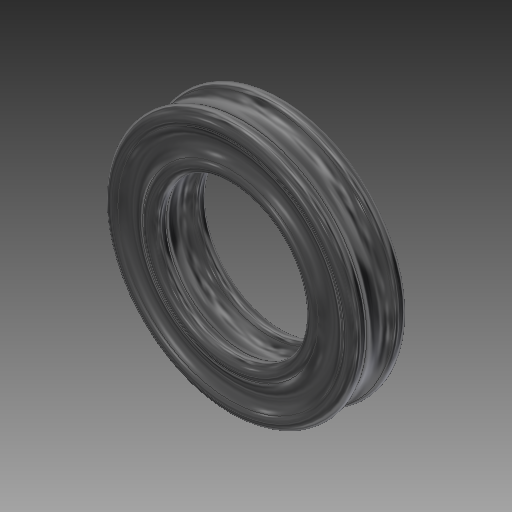
# Autodesk Inventor part: X-Ring 6x2.6
Saved by Autodesk Inventor 2017.3 (Build 213256000, 256)
## iProperties
Created: 2015-08-15
Part Number: X-Ring 6x2.6
Material: Gummi, Silikon
Document SubType Name: Modeling
Designer: rYan
Mass: 0.187427 g
Surface Area: 3.05947 cm^2
Volume: 0.149942 cm^3
Density: 1.25 g/cm^3
Appearance: Gummi - schwarz - Version 1.1
Author: rYan
Autodesk Inventor part; units mm, degrees
ref_plane "YZ Plane" through (0, 0, 0) normal (1, 0, 0) x (0, 1, 0)
ref_plane "XZ Plane" through (0, 0, 0) normal (0, 1, 0) x (-1, 0, 0)
ref_plane "XY Plane" through (0, 0, 0) normal (0, 0, 1) x (1, 0, 0)
sketch "Skizze1" plane through (0, 0, 0) normal (1, 0, 0) x (0, 1, 0)
  arc A0 (-0.63, 5.8857) -> (-1.2127, 5.3385) centre (-0.91, 5.6) ccw
  arc A1 (-0.63, 5.8857) -> (0.63, 5.8857) centre (0, 6.5284) ccw
  arc A2 (1.2127, 5.3385) -> (0.63, 5.8857) centre (0.91, 5.6) ccw
  arc A3 (1.2127, 5.3385) -> (1.2127, 4.1615) centre (1.8936, 4.75) ccw
  arc A4 (0.63, 3.6143) -> (1.2127, 4.1615) centre (0.91, 3.9) ccw
  arc A5 (0.63, 3.6143) -> (-0.63, 3.6143) centre (0, 2.9716) ccw
  arc A6 (-1.2127, 4.1615) -> (-0.63, 3.6143) centre (-0.91, 3.9) ccw
  arc A7 (-1.2127, 4.1615) -> (-1.2127, 5.3385) centre (-1.8936, 4.75) ccw
  line L0 (-0.91, 5.6) -> (0.91, 5.6) construction
  line L1 (0.91, 5.6) -> (0.91, 3.9) construction
  line L2 (0.91, 3.9) -> (-0.91, 3.9) construction
  line L3 (-0.91, 3.9) -> (-0.91, 5.6) construction
  line L4 (0, 7.8341) -> (0, -1.3057) projected
  line L5 (-2.6511, 0) -> (2.6511, 0) construction
  line L6 (0, 5.6) -> (0, 3.9) construction
  line L7 (-0.91, 4.75) -> (0.91, 4.75) construction
  line L8 (-0.91, 5.6) -> (-1.31, 5.6) construction
  line L9 (-0.91, 3.9) -> (-1.31, 3.9) construction
  line L10 (-1.31, 3.9) -> (-1.31, 5.6) construction
  line L11 (-0.91, 5.6) -> (-0.91, 6) construction
  line L12 (-0.91, 3.9) -> (-0.91, 3.5) construction
  line L13 (0.91, 3.9) -> (0.91, 3.5) construction
  line L14 (-0.91, 3.5) -> (0.91, 3.5) construction
  line L15 (0.91, 5.6) -> (1.31, 5.6) construction
  line L16 (0.91, 3.9) -> (1.31, 3.9) construction
  line L17 (-0.91, 6) -> (0.91, 6) construction
  point P0 (0, 0)
  dimension "d0" = 2.5
  dimension "d1" = 7
  dimension "d2" = 2.62
  dimension "d3" = 0.9
  dimension "d4" = 0.4
  constraints: 32 end point, 25 point on circle, 10 tangent, 8 centre point, 7 parallel, 4 horizontal, 4 midpoint, 2 equal radius, 2 vertical, 1 point on line, 3 other
  measures "d0" distance of L12.end L11.end
  measures "d1" diameter of L14 L5
  measures "d2" distance of L8.end L15.end
  measures "d3" radius of A7
  measures "d4" radius of A0
revolve "Umdrehung1" add sketch "Skizze1" angle 360 about axis through (0, 0, 0) along (0, 1, 0)
